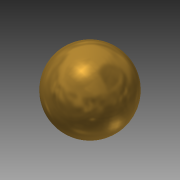
# Autodesk Inventor part: ball bearing .5in
Saved by Autodesk Inventor 2015 SP2 (Build 190223200, 223)
## iProperties
Created: 2015-05-24
Part Number: ball bearing .5in
Material: Generic
Document SubType Name: Modeling
Designer: caleb
Density: 1 g/cm^3
Appearance: Default
Author: caleb
Autodesk Inventor part; units mm, degrees
ref_plane "YZ Plane" through (0, 0, 0) normal (1, 0, 0) x (0, 1, 0)
ref_plane "XZ Plane" through (0, 0, 0) normal (0, 1, 0) x (-1, 0, 0)
ref_plane "XY Plane" through (0, 0, 0) normal (0, 0, 1) x (1, 0, 0)
sketch "Sketch1" plane through (0, 0, 0) normal (0, 0, 1) x (1, 0, 0)
  arc A0 (6.35, 0) -> (-6.35, 0) centre (0, 0) ccw
  line L0 (-6.35, 0) -> (6.35, 0)
  point P0 (0, 0)
  dimension "d0" = 6.35
  constraints: 2 coincident, 2 end point, 2 point on circle, 1 centre point, 1 horizontal, 1 midpoint
  measures "d0" radius of A0
revolve "Revolution1" add sketch "Sketch1" angle 360 about axis through (-6.35, 0, 0) along (1, 0, 0)
body "Solid1"
